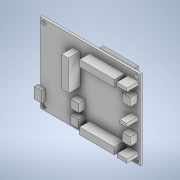
# Autodesk Inventor part: lunchpad
Saved by Autodesk Inventor 2022 (Build 260153000, 153)
## iProperties
Created: 2021-08-24
Part Number: lunchpad
Material: Generic
Document SubType Name: Modeling
Designer: jonar
Density: 1 g/cm^3
Appearance: Default
Author: jonar
Autodesk Inventor part; units mm, degrees
ref_plane "YZ Plane" through (0, 0, 0) normal (1, 0, 0) x (0, 1, 0)
ref_plane "XZ Plane" through (0, 0, 0) normal (0, 1, 0) x (-1, 0, 0)
ref_plane "XY Plane" through (0, 0, 0) normal (0, 0, 1) x (1, 0, 0)
sketch "card" plane through (0, 0, 0) normal (0, 0, 1) x (1, 0, 0)
  line L0 (-59.3579, 68.5808) -> (-59.3579, 10.0008)
  line L1 (-59.3579, 10.0008) -> (14.2921, 10.0008)
  line L2 (14.2921, 10.0008) -> (14.2921, 68.5808)
  line L3 (14.2921, 68.5808) -> (-59.3579, 68.5808)
  circle A0 centre (11.6671, 65.9558) radius 1.575
  circle A1 centre (11.6671, 12.6258) radius 1.575
  circle A2 centre (-56.7329, 65.9558) radius 1.575
  circle A3 centre (-56.7329, 12.6258) radius 1.575
  point P0 (0, 0)
  dimension "d1" = 58.58
  dimension "d2" = 73.65
  dimension "d4" = 2.625
  dimension "d5" = 3.15
  constraints: 8 end point, 4 centre point, 2 perpendicular, 1 vertical
  measures "d1" distance of L1.end L2.end
  measures "d2" distance of L2.end L0.start
  measures "d4" distance from line of L2 A0.centre
  measures "d5" diameter of A0
extrude "main_board" add sketch "card" along normal blind 1.6
sketch "back_components" plane through (0, 0, 0) normal (0, 0, -1) x (-1, 0, 0)
  line L0 (-3.0921, 63.3708) -> (22.7279, 63.3708)
  line L1 (22.7279, 63.3708) -> (22.7279, 58.3708)
  line L2 (22.7279, 58.3708) -> (-3.0921, 58.3708)
  line L3 (-3.0921, 58.3708) -> (-3.0921, 63.3708)
  line L4 (-2.9921, 20.1008) -> (22.8179, 20.1008)
  line L5 (22.8179, 20.1008) -> (22.8179, 15.1008)
  line L6 (22.8179, 15.1008) -> (-2.9921, 15.1008)
  line L7 (-2.9921, 15.1008) -> (-2.9921, 20.1008)
  line L8 (-14.2921, 68.5808) -> (59.3579, 68.5808) projected
  line L9 (-14.2921, 10.0008) -> (-14.2921, 68.5808) projected
  line L10 (59.3579, 10.0008) -> (-14.2921, 10.0008) projected
  point P0 (0, 0)
  dimension "d23" = 5.21
  dimension "d24" = 11.2
  dimension "d25" = 5.1
  dimension "d26" = 11.3
  dimension "d27" = 5
  dimension "d28" = 5
  dimension "d29" = 25.82
  dimension "d30" = 25.81
  constraints: 16 end point, 3 parallel, 2 horizontal, 2 perpendicular
  measures "d23" distance between parallel lines of L8 L0
  measures "d24" distance between parallel lines of L9 L3
  measures "d25" distance between parallel lines of L10 L6
  measures "d26" distance between parallel lines of L9 L7
  measures "d27" distance between parallel lines of L6 L4
  measures "d28" distance between parallel lines of L0 L2
  measures "d29" distance between parallel lines of L1 L3
  measures "d30" distance between parallel lines of L5 L7
extrude "pins_female" add sketch "back_components" along normal blind 8.37
extrude "pins_male1" add sketch "back_components" against normal blind 9.24 contours L0 L1 L2 L3
extrude "pins_male2" add sketch "back_components" against normal blind 9.24
sketch "front_components" plane through (0, 0, 1.6) normal (0, 0, 1) x (1, 0, 0)
  line L0 (-55.4979, 24.5008) -> (-61.1579, 24.5008)
  line L1 (-61.1579, 24.5008) -> (-61.1579, 16.5008)
  line L2 (-61.1579, 16.5008) -> (-55.4979, 16.5008)
  line L3 (-55.4979, 16.5008) -> (-55.4979, 24.5008)
  line L4 (-59.3579, 10.0008) -> (14.2921, 10.0008) projected
  line L5 (-59.3579, 68.5808) -> (-59.3579, 10.0008) projected
  line L6 (-35.1979, 60.9808) -> (-30.0979, 60.9808)
  line L7 (-30.0979, 60.9808) -> (-30.0979, 38.4308)
  line L8 (-30.0979, 38.4308) -> (-35.1979, 38.4308)
  line L9 (-35.1979, 38.4308) -> (-35.1979, 60.9808)
  line L10 (-32.0779, 22.0008) -> (-26.0779, 22.0008)
  line L11 (-26.0779, 22.0008) -> (-26.0779, 16.0008)
  line L12 (-26.0779, 16.0008) -> (-32.0779, 16.0008)
  line L13 (-32.0779, 16.0008) -> (-32.0779, 22.0008)
  line L14 (-22, 22) -> (-2, 22)
  line L15 (-2, 22) -> (-2, 16)
  line L16 (-2, 16) -> (-22, 16)
  line L17 (-22, 16) -> (-22, 22)
  line L18 (5.8421, 17.9408) -> (13.1421, 17.9408)
  line L19 (13.1421, 17.9408) -> (13.1421, 15.3408)
  line L20 (13.1421, 15.3408) -> (5.8421, 15.3408)
  line L21 (5.8421, 15.3408) -> (5.8421, 17.9408)
  line L22 (6.0921, 29.8608) -> (12.0921, 29.8608)
  line L23 (12.0921, 29.8608) -> (12.0921, 23.8608)
  line L24 (12.0921, 23.8608) -> (6.0921, 23.8608)
  line L25 (6.0921, 23.8608) -> (6.0921, 29.8608)
  line L26 (7.8321, 40.7108) -> (12.8321, 40.7108)
  line L27 (12.8321, 40.7108) -> (12.8321, 38.2308)
  line L28 (12.8321, 38.2308) -> (7.8321, 38.2308)
  line L29 (7.8321, 38.2308) -> (7.8321, 40.7108)
  line L30 (6.0921, 55.0808) -> (12.0921, 55.0808)
  line L31 (12.0921, 55.0808) -> (12.0921, 49.0808)
  line L32 (12.0921, 49.0808) -> (6.0921, 49.0808)
  line L33 (6.0921, 49.0808) -> (6.0921, 55.0808)
  line L34 (5.6421, 63.4208) -> (13.1421, 63.4208)
  line L35 (13.1421, 63.4208) -> (13.1421, 60.9408)
  line L36 (13.1421, 60.9408) -> (5.6421, 60.9408)
  line L37 (5.6421, 60.9408) -> (5.6421, 63.4208)
  line L38 (-27, 66) -> (-6, 66)
  line L39 (-6, 66) -> (-6, 62)
  line L40 (-6, 62) -> (-27, 62)
  line L41 (-27, 62) -> (-27, 66)
  line L42 (-32.0779, 26.1508) -> (-26.0779, 26.1508)
  line L43 (-26.0779, 26.1508) -> (-26.0779, 32.1508)
  line L44 (-26.0779, 32.1508) -> (-32.0779, 32.1508)
  line L45 (-32.0779, 32.1508) -> (-32.0779, 26.1508)
  line L46 (14.2921, 68.5808) -> (-59.3579, 68.5808) projected
  line L47 (14.2921, 10.0008) -> (14.2921, 68.5808) projected
  point P0 (0, 0)
  dimension "d19" = 6.5
  dimension "d20" = 8
  dimension "d21" = 1.8
  dimension "d22" = 5.66
  dimension "d31" = 27.28
  dimension "d32" = 6
  dimension "d33" = 6
  dimension "d34" = 6
  dimension "d35" = 4.15
  dimension "d36" = 6
  dimension "d37" = 6
  dimension "d38" = 5.16
  dimension "d39" = 2.48
  dimension "d40" = 5.86
  dimension "d41" = 6
  dimension "d42" = 6
  dimension "d43" = 8.37
  dimension "d44" = 2.48
  dimension "d45" = 7.5
  dimension "d46" = 6
  dimension "d47" = 6
  dimension "d48" = 8.37
  dimension "d49" = 5.92
  dimension "d50" = 2.6
  dimension "d51" = 1.15
  dimension "d58" = 7.6
  dimension "d59" = 22.55
  dimension "d60" = 5.1
  dimension "d61" = 24.16
  dimension "d62" = 2.2
  dimension "d63" = 1.46
  dimension "d64" = 5
  dimension "d65" = 7.3
  dimension "d66" = 1.15
  constraints: 88 end point, 20 parallel, 12 perpendicular, 11 horizontal, 2 collinear, 1 vertical
  measures "d19" distance between parallel lines of L2 L4
  measures "d20" distance between parallel lines of L0 L2
  measures "d21" distance between parallel lines of L5 L1
  measures "d22" distance between parallel lines of L3 L1
  measures "d31" distance between parallel lines of L5 L13
  measures "d32" distance between parallel lines of L11 L13
  measures "d33" distance between parallel lines of L12 L10
  measures "d34" distance between parallel lines of L12 L4
  measures "d35" distance between parallel lines of L42 L10
  measures "d36" distance between parallel lines of L44 L42
  measures "d37" distance between parallel lines of L43 L45
  measures "d38" distance between parallel lines of L46 L34
  measures "d39" distance between parallel lines of L34 L36
  measures "d40" distance between parallel lines of L36 L30
  measures "d41" distance between parallel lines of L30 L32
  measures "d42" distance between parallel lines of L33 L31
  measures "d43" distance between parallel lines of L32 L26
  measures "d44" distance between parallel lines of L26 L28
  measures "d45" distance between parallel lines of L35 L37
  measures "d46" distance between parallel lines of L23 L25
  measures "d47" distance between parallel lines of L22 L24
  measures "d48" distance between parallel lines of L22 L28
  measures "d49" distance between parallel lines of L24 L18
  measures "d50" distance between parallel lines of L20 L18
  measures "d51" distance from line of L47 L34.end
  measures "d58" distance between parallel lines of L46 L6
  measures "d59" distance between parallel lines of L6 L8
  measures "d60" distance between parallel lines of L7 L9
  measures "d61" distance between parallel lines of L5 L9
  measures "d62" distance between parallel lines of L47 L23
  measures "d63" distance between parallel lines of L47 L27
  measures "d64" distance between parallel lines of L29 L27
  measures "d65" distance between parallel lines of L21 L19
  measures "d66" distance between parallel lines of L47 L19
extrude "vcc_gnd" add sketch "front_components" along normal blind 8.53 contours L18 L19 L20 L21 | L34 L35 L36 L37
extrude "buttons" add sketch "front_components" along normal blind 5 contours L10 L11 L12 L13 | L22 L23 L24 L25 | L30 L31 L32 L33 | L45 L44 L43 L42
extrude "sikring" add sketch "front_components" along normal blind 8.5 contours L6 L7 L8 L9 | L26 L27 L28 L29
extrude "Extrusion8" add sketch "front_components" along normal blind 2.8 contours L3 L2 L5 L0 | L5 L2 L1 L0
body "Solid1"
